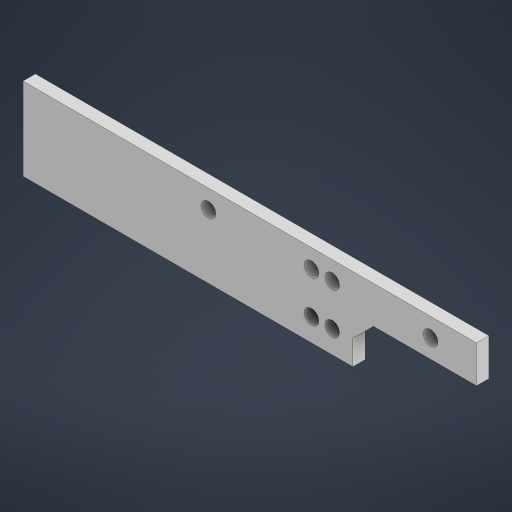
# Autodesk Inventor part: Slide_Climb_Hook_Mounts
Saved by Autodesk Inventor 2023 (Build 270158000, 158)
## iProperties
Created: 2024-02-27
Part Number: Slide_Climb_Hook_Mounts
Material: Generic
Document SubType Name: Modeling
Designer: kelle
Density: 1 g/cm^3
Appearance: Default
Mass: 13.8932 g
Surface Area: 93.4773 cm^2
Volume: 13.8932 cm^3
Author: kelle
Autodesk Inventor part; units mm, degrees
ref_plane "YZ Plane" through (0, 0, 0) normal (1, 0, 0) x (0, 1, 0)
ref_plane "XZ Plane" through (0, 0, 0) normal (0, 1, 0) x (-1, 0, 0)
ref_plane "XY Plane" through (0, 0, 0) normal (0, 0, 1) x (1, 0, 0)
sketch "Sketch1" plane through (0, 0, 0) normal (0, 0, 1) x (1, 0, 0)
  line L0 (76.2, -5.715) -> (-76.2, -5.715)
  line L1 (-76.2, -5.715) -> (-76.2, 5.715)
  line L2 (-76.2, 5.715) -> (76.2, 5.715)
  line L3 (76.2, 5.715) -> (76.2, -5.715)
  line L4 (76.2, -5.715) -> (-76.2, 5.715) construction
  line L5 (-76.2, -5.715) -> (76.2, 5.715) construction
  circle A0 centre (-6.35, 0) radius 2.25
  circle A1 centre (62.0522, 0) radius 2.25
  circle A2 centre (25.4, 0) radius 2.25
  circle A3 centre (31.75, 0) radius 2.25
  circle A4 centre (25.4, -12.7) radius 2.25
  circle A5 centre (31.75, -12.7) radius 2.25
  line L6 (0, 5.715) -> (-76.2, 5.715)
  line L7 (38.1, 5.715) -> (-63.5, 5.715)
  line L8 (-63.5, 5.715) -> (-63.5, -19.685)
  line L9 (-63.5, -19.685) -> (38.1, -19.685)
  line L10 (38.1, -19.685) -> (38.1, 5.715)
  point P0 (0, 0)
  point P1 (38.1, -5.715)
  point P2 (-63.5, -5.715)
  dimension "d0" = 152.4
  dimension "d1" = 11.43
  dimension "d2" = 4.5
  dimension "d3" = 4.5
  dimension "d4" = 68.4022
  dimension "d5" = 69.85
  dimension "d6" = 4.5
  dimension "d9" = 101.6
  dimension "d12" = 6.35
  dimension "d15" = 12.7
  dimension "d22" = 101.6
  dimension "d23" = 25.4
  dimension "d24" = 6.35
  constraints: 22 end point, 6 centre point, 4 horizontal, 4 parallel, 3 midpoint, 2 perpendicular, 1 point on line, 1 vertical, 6 other
  measures "d0" distance of L1.end L2.end
  measures "d1" distance of L0.end L1.end
  measures "d2" diameter of A0
  measures "d3" diameter of A1
  measures "d4" distance of A0.centre A1.centre
  measures "d5" distance from line of L1 A0.centre
  measures "d6" diameter of A2
  measures "d9" distance from line of L1 A2.centre
  measures "d12" distance of A2.centre A3.centre
  measures "d15" distance of A2.centre A4.centre
  measures "d22" distance of L9.end L8.end
  measures "d23" distance of L8.end L7.end
  measures "d24" distance from line of A3.centre L10
extrude "Extrusion1" add sketch "Sketch1" along normal blind 3.81
fillet "Fillet1" [suppressed]
sketch "Sketch2" plane through (0, 0, 3.81) normal (0, 0, 1) x (1, 0, 0)
  line L0 (76.2, 5.715) -> (-76.2, 5.715) projected
  line L1 (-76.2, 5.715) -> (-76.2, -5.715) projected
  line L2 (-76.2, -5.715) -> (-63.5, -5.715) projected
  line L3 (-63.5, -5.715) -> (-63.5, -19.685) projected
  line L4 (-63.5, -19.685) -> (38.1, -19.685) projected
  line L5 (38.1, -19.685) -> (38.1, -5.715) projected
  line L6 (38.1, -5.715) -> (76.2, -5.715) projected
  line L7 (76.2, -5.715) -> (76.2, 5.715) projected
  circle A0 centre (-6.35, 0) radius 2.25 projected
  circle A1 centre (62.0522, 0) radius 2.25 projected
  circle A2 centre (25.4, 0) radius 2.25 projected
  circle A3 centre (31.75, 0) radius 2.25 projected
  circle A4 centre (31.75, -12.7) radius 2.25 projected
  circle A5 centre (25.4, -12.7) radius 2.25 projected
  line L8 (-63.5, -5.715) -> (-76.2, -5.715)
  line L9 (-76.2, -5.715) -> (-76.2, 5.715)
  line L10 (-76.2, 5.715) -> (-63.5, 5.715)
  line L11 (-63.5, 5.715) -> (-63.5, -5.715)
  point P0 (0, 0)
  constraints: 8 end point, 2 parallel, 1 horizontal, 1 perpendicular
extrude "Extrusion2" cut sketch "Sketch2" against normal through all contours L11 L2 L1 L0
chamfer "Chamfer1" distance 6.35 angle 45 1 edges at (38.1, -5.715, 1.905)
body "Solid1"
